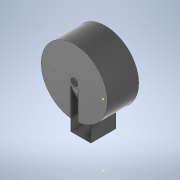
# Autodesk Inventor part: Grundplatte
Saved by Autodesk Inventor 2020.3 (Build 243373000, 373)
## iProperties
Created: 2021-08-11
Part Number: Grundplatte
Material: Acetalharz, Schwarz
Document SubType Name: Modeling
Designer: Preuß P. Ch.
Density: 1.425 g/cm^3
Appearance: Glatt - Schwarz
Author: Preuß P. Ch.
Autodesk Inventor part; units mm, degrees
ref_plane "YZ Plane" through (0, 0, 0) normal (1, 0, 0) x (0, 1, 0)
ref_plane "XZ Plane" through (0, 0, 0) normal (0, 1, 0) x (-1, 0, 0)
ref_plane "XY Plane" through (0, 0, 0) normal (0, 0, 1) x (1, 0, 0)
sketch "Skizze1" plane through (0, 0, 0) normal (0, 1, 0) x (-1, 0, 0)
  line L0 (2000, 0) -> (-2000, 0)
  line L1 (-2000, 0) -> (-2000, -10)
  line L2 (-2000, -10) -> (2000, -10)
  line L3 (2000, -10) -> (2000, 0)
  dimension "d3" = 4000
  dimension "d4" = 10
  constraints: 8 end point, 2 parallel, 1 horizontal, 1 perpendicular
  measures "d3" distance of L2.end L1.end
  measures "d4" distance of L1.end L0.end
extrude "Extrusion1" add sketch "Skizze1" along normal mid plane 4000
sketch "Skizze2" plane through (-2000, 2000, 0) normal (0, 0, 1) x (1, 0, 0)
  line L0 (20, -1975) -> (433.5, -1975)
  line L1 (433.5, -1975) -> (433.5, -2025)
  line L2 (433.5, -2025) -> (20, -2025)
  line L3 (20, -2025) -> (20, -1975)
  circle A0 centre (433.5, -1975) radius 5
  circle A1 centre (433.5, -2025) radius 5
  circle A2 centre (20, -2025) radius 5
  circle A3 centre (20, -1975) radius 5
  point P0 (2000, -2000)
  dimension "d7" = 413.5
  dimension "d8" = 50
  dimension "d9" = 10
  dimension "d10" = 10
  dimension "d11" = 10
  dimension "d12" = 10
  constraints: 8 end point, 4 centre point, 4 coincident, 2 parallel, 1 horizontal, 1 perpendicular
  measures "d7" distance of L1.end L2.end
  measures "d8" distance of L0.end L1.end
  measures "d9" diameter of A0
  measures "d10" diameter of A1
  measures "d11" diameter of A2
  measures "d12" diameter of A3
hole "Bohrung1" at (-1566.5, 25, 0) at (-1566.5, -25, 0) at (-1980, -25, 0) at (-1980, 25, 0) direction (0, 0, -1) diameter 6.647 depth 10 tip angle 118 thread size "M8x1.25" class "6H" standard "ISO Metric profile"
chamfer "Fase1" distance 1 angle 45 4 edges at (-1980, 28.3235, 0) (-1980, -21.6765, 0) (-1566.5, 28.3235, 0) (-1566.5, -21.6765, 0)
sketch "Skizze3" plane through (-2000, 2000, 0) normal (0, 0, 1) x (1, 0, 0)
  circle A0 centre (1065, -2000) radius 105
  point P0 (2000, -2000)
  dimension "d23" = 210
  constraints: 1 centre point
  measures "d23" diameter of A0
extrude "Extrusion2" cut sketch "Skizze3" against normal blind 10
chamfer "Fase2" distance 10 angle 45 1 edges at (-1040, 0, 0)
sketch "Skizze4" plane through (-2000, 2000, 0) normal (0, 0, 1) x (1, 0, 0)
  line L0 (1090, -2000) -> (1040, -2000)
  line L1 (1040, -2000) -> (1040, -1555.368)
  line L2 (1040, -1555.368) -> (1090, -1555.368)
  line L3 (1090, -1555.368) -> (1090, -2000)
  line L4 (1090, -1555.368) -> (1040, -1555.368)
  line L5 (1040, -1555.368) -> (1040, -1141.868)
  line L6 (1040, -1141.868) -> (1090, -1141.868)
  line L7 (1090, -1141.868) -> (1090, -1555.368)
  point P0 (2000, -2000)
  dimension "d29" = 50
  dimension "d30" = 444.632
  dimension "d31" = 413.5
  constraints: 16 end point, 4 parallel, 2 horizontal, 2 perpendicular, 1 point on line
  measures "d29" distance of L1.end L2.end
  measures "d30" distance of L0.end L1.end
  measures "d31" distance of L4.end L5.end
hole "Bohrung2" at (-960, 444.632, 0) at (-910, 444.632, 0) at (-960, 858.132, 0) at (-910, 858.132, 0) direction (0, 0, -1) diameter 6.647 depth 10 tip angle 118 thread size "M8x1.25" class "6H" standard "ISO Metric profile"
fillet "Rundung1" radius 0.5 1 edges at (-960, 447.9555, 0)
sketch "Skizze5" plane through (-2000, 2000, 0) normal (0, 0, 1) x (1, 0, 0)
  circle A0 centre (1065, -2000) radius 115 projected
  line L0 (715, -2155) -> (945, -2155)
  line L1 (945, -2155) -> (945, -1845)
  line L2 (945, -1845) -> (715, -1845)
  line L3 (715, -1845) -> (715, -2155)
  line L4 (715, -1845) -> (735, -1845)
  line L5 (735, -1845) -> (735, -1865)
  line L6 (735, -1865) -> (715, -1865)
  line L7 (715, -1865) -> (715, -1845)
  line L8 (945, -1845) -> (925, -1845)
  line L9 (925, -1845) -> (925, -1865)
  line L10 (925, -1865) -> (945, -1865)
  line L11 (945, -1865) -> (945, -1845)
  line L12 (945, -2155) -> (925, -2155)
  line L13 (925, -2155) -> (925, -2135)
  line L14 (925, -2135) -> (945, -2135)
  line L15 (945, -2135) -> (945, -2155)
  line L16 (715, -2155) -> (735, -2155)
  line L17 (735, -2155) -> (735, -2135)
  line L18 (735, -2135) -> (715, -2135)
  line L19 (715, -2135) -> (715, -2155)
  point P0 (2000, -2000)
  dimension "d43" = 230
  dimension "d44" = 310
  dimension "d45" = 20
  dimension "d46" = 20
  dimension "d47" = 20
  dimension "d48" = 20
  dimension "d49" = 20
  dimension "d50" = 20
  dimension "d51" = 20
  constraints: 40 end point, 10 parallel, 5 horizontal, 5 perpendicular, 1 point on line
  measures "d43" distance of L2.end L1.end
  measures "d44" distance of L1.end L0.end
  measures "d45" distance of L5.end L6.end
  measures "d46" distance of L4.end L5.end
  measures "d47" distance of L10.end L9.end
  measures "d48" distance of L13.end L14.end
  measures "d49" distance of L12.end L13.end
  measures "d50" distance of L18.end L17.end
  measures "d51" distance of L17.end L16.end
hole "Bohrung3" at (-1265, -135, 0) at (-1265, 135, 0) at (-1075, -135, 0) at (-1075, 135, 0) direction (0, 0, -1) diameter 8.376 depth 27.3 tip angle 118 thread size "M10x1.5" class "6H" standard "ISO Metric profile"
sketch "Skizze9" plane through (2000, 2000, -10) normal (0, 0, -1) x (-1, 0, 0)
  circle A0 centre (2935, -2000) radius 105 projected
  line L0 (2780, -2000) -> (2780, -2155)
  line L1 (2780, -2155) -> (2935, -2155)
  line L2 (2780, -2155) -> (3090, -2155)
  line L3 (3090, -2155) -> (3090, -1845)
  line L4 (3090, -1845) -> (2780, -1845)
  line L5 (2780, -1845) -> (2780, -2155)
  line L6 (2780, -2155) -> (2795, -2155)
  line L7 (2795, -2155) -> (2795, -2135)
  line L8 (2795, -2135) -> (2780, -2135)
  line L9 (2780, -2135) -> (2780, -2155)
  line L10 (2780, -1845) -> (2795, -1845)
  line L11 (2795, -1845) -> (2795, -1865)
  line L12 (2795, -1865) -> (2780, -1865)
  line L13 (2780, -1865) -> (2780, -1845)
  point P0 (2000, -2000)
  dimension "d73" = 155
  dimension "d74" = 310
  dimension "d75" = 310
  dimension "d76" = 15
  dimension "d77" = 20
  dimension "d78" = 20
  constraints: 28 end point, 6 parallel, 3 horizontal, 3 perpendicular, 1 point on line
  measures "d73" distance of L1.end L0.end
  measures "d74" distance of L4.end L3.end
  measures "d75" distance of L3.end L2.end
  measures "d76" distance of L8.end L7.end
  measures "d77" distance of L7.end L6.end
  measures "d78" distance of L10.end L11.end
hole "Bohrung4" at (-795, -135, -10) at (-795, 135, -10) direction (0, 0, 1) diameter 8.376 depth 27.3 tip angle 118 thread size "M10x1.5" class "6H" standard "ISO Metric profile"
chamfer "Fase3" distance 4 angle 45 2 edges at (-795, -139.188, 0) (-795, 130.812, 0)
sketch "Skizze10" plane through (-2000, 2000, 0) normal (0, 0, 1) x (1, 0, 0)
  line L0 (0, 0) -> (4000, 0) projected
  line L1 (1185, -2155) -> (943, -2155)
  line L2 (943, -2155) -> (943, -3077.5)
  line L3 (943, -3077.5) -> (1185, -3077.5)
  line L4 (1185, -3077.5) -> (1185, -2155)
  point P0 (2000, -2000)
  dimension "d92" = 242
  dimension "d93" = 922.5
  constraints: 8 end point, 2 parallel, 1 horizontal, 1 perpendicular
  measures "d92" distance of L3.end L2.end
  measures "d93" distance of L2.end L1.end
extrude "Extrusion6" cut sketch "Skizze10" against normal blind 10
sketch "Skizze11" plane through (2000, 2000, -10) normal (0, 0, -1) x (-1, 0, 0)
  line L0 (3057, -3077.5) -> (3057, -2155) projected
  line L1 (3057, -3077.5) -> (3067, -3077.5)
  line L2 (3067, -3077.5) -> (3067, -2827.5)
  line L3 (3067, -2827.5) -> (3057, -2827.5)
  line L4 (3057, -2827.5) -> (3057, -3077.5)
  line L5 (2815, -3077.5) -> (2815, -2155) projected
  line L6 (2815, -3077.5) -> (2805, -3077.5)
  line L7 (2805, -3077.5) -> (2805, -2827.5)
  line L8 (2805, -2827.5) -> (2815, -2827.5)
  line L9 (2815, -2827.5) -> (2815, -3077.5)
  line L10 (3067, -3077.5) -> (2805, -3077.5)
  line L11 (2805, -3077.5) -> (2805, -3087.5)
  line L12 (2805, -3087.5) -> (3067, -3087.5)
  line L13 (3067, -3087.5) -> (3067, -3077.5)
  point P0 (2000, -2000)
  dimension "d96" = 10
  dimension "d97" = 250
  dimension "d98" = 10
  dimension "d99" = 250
  dimension "d100" = 10
  constraints: 24 end point, 6 parallel, 3 horizontal, 3 perpendicular, 1 point on line
  measures "d96" distance of L3.end L2.end
  measures "d97" distance of L2.end L1.end
  measures "d98" distance of L7.end L8.end
  measures "d99" distance of L6.end L7.end
  measures "d100" distance of L11.end L10.end
extrude "Extrusion7" add sketch "Skizze11" along normal blind 400
sketch "Skizze12" plane through (2000, 2000, -410) normal (0, 0, -1) x (-1, 0, 0)
  line L0 (3067, -3087.5) -> (2805, -3087.5) projected
  line L1 (2805, -2827.5) -> (2805, -3087.5) projected
  line L2 (3067, -3087.5) -> (2805, -3087.5)
  line L3 (2805, -3087.5) -> (2805, -2827.5)
  line L4 (2805, -2827.5) -> (3067, -2827.5)
  line L5 (3067, -2827.5) -> (3067, -3087.5)
  point P0 (2000, -2000)
  constraints: 8 end point, 2 parallel, 1 horizontal, 1 perpendicular
extrude "Extrusion8" add sketch "Skizze12" along normal blind 10
sketch "Skizze13" plane through (-1057, -827.5, -410) normal (0, 1, 0) x (1, 0, 0)
  line L0 (252, 10) -> (-10, 10) projected
  line L1 (252, -400) -> (252, 10) projected
  line L2 (-10, 10) -> (252, 10)
  line L3 (252, 10) -> (252, -140)
  line L4 (252, -140) -> (-10, -140)
  line L5 (-10, -140) -> (-10, 10)
  point P0 (1057, -410)
  dimension "d105" = 150
  constraints: 8 end point, 2 parallel, 1 horizontal, 1 perpendicular, 1 point on line
  measures "d105" distance of L2.end L3.end
extrude "Extrusion9" add sketch "Skizze13" along normal blind 10
sketch "Skizze14" plane through (-1067, -1087.5, -10) normal (-1, 0, 0) x (0, 0, 1)
  line L0 (0, 260) -> (0, 932.5) projected
  line L1 (-260, 270) -> (0, 932.5)
  line L2 (0, 932.5) -> (0, 260)
  line L3 (0, 260) -> (-260, 260)
  line L4 (-260, 260) -> (-260, 270)
  point P0 (10, 1087.5)
  constraints: 8 end point, 2 perpendicular, 1 collinear
extrude "Extrusion10" add sketch "Skizze14" against normal blind 10
sketch "Skizze15" plane through (-805, -1087.5, -10) normal (1, 0, 0) x (0, 0, -1)
  line L0 (410, 270) -> (260, 270) projected
  line L1 (0, 932.5) -> (260, 270) projected
  line L2 (260, 270) -> (0, 932.5)
  line L3 (0, 260) -> (260, 260) projected
  line L4 (0, 932.5) -> (0, 260)
  line L5 (0, 260) -> (260, 260)
  line L6 (260, 270) -> (260, 260) projected
  line L7 (260, 260) -> (260, 270)
  point P0 (-10, 1087.5)
  constraints: 8 end point, 2 collinear, 1 perpendicular
extrude "Extrusion11" add sketch "Skizze15" against normal blind 10
sketch "Skizze16" plane through (-805, -817.5, -270) normal (0, 0.3653263, -0.9308795) x (-1, 0, 0)
  line L0 (0, 0) -> (0, 711.692525)
  line L1 (262, 711.692525) -> (262, 0)
  line L2 (0, 0) -> (262, 0)
  line L3 (262, 0) -> (262, 711.692525)
  line L4 (262, 711.692525) -> (0, 711.692525)
  line L5 (0, 711.692525) -> (0, 0)
  point P0 (-805, 859.632114)
  constraints: 8 end point, 2 parallel, 1 horizontal, 1 perpendicular
extrude "Extrusion12" add sketch "Skizze16" along normal blind 10
sketch "Skizze17" plane through (-2000, 2000, 0) normal (0, 0, 1) x (1, 0, 0)
  point P0 (2000, -2000)
sketch "Skizze18" plane through (0, -2000, 0) normal (0, -1, 0) x (1, 0, 0)
  point P0 (0, 0)
sketch "Skizze19" plane through (0, -2000, 0) normal (0, -1, 0) x (1, 0, 0)
  point P0 (0, 0)
sketch "Skizze20" plane through (2000, 2000, -10) normal (0, 0, -1) x (-1, 0, 0)
  circle A0 centre (3075, -1865) radius 4.188
  line L0 (3075, -1865) -> (2935, -1865)
  line L1 (2935, -1865) -> (2935, -2000)
  line L2 (2935, -2000) -> (3075, -2000)
  line L3 (3075, -2000) -> (3075, -1865)
  circle A1 centre (2935, -2000) radius 612.5
  circle A2 centre (2935, -2000) radius 1065
  line L4 (2805, -2151.346737) -> (2805, -2813.846737)
  line L5 (3067, -2155) -> (3067, -3087.5)
  line L6 (2805, -2598.545111) -> (3067, -2598.545111)
  line L7 (3067, -2598.545111) -> (3067, -3087.5)
  line L8 (3067, -3087.5) -> (2805, -3087.5)
  line L9 (2805, -3087.5) -> (2805, -2598.545111)
  point P0 (2000, -2000)
  point P1 (2805, -3057.03595)
  point P2 (3067, -2598.107223)
  point P3 (3067, -3056.788058)
  dimension "d117" = 1225
  dimension "d114" = 140
  dimension "d115" = 135
  constraints: 16 end point, 4 parallel, 2 horizontal, 2 perpendicular, 1 centre point, 1 coincident, 1 point on line, 3 other
  measures "d114" distance of L2.end L1.end
  measures "d115" distance of L1.end L0.end
extrude "Extrusion13" add sketch "Skizze20" along normal blind 1000 contours A1 L4 L9 A2 L5
sketch "Skizze21" plane through (2000, 2000, -420) normal (0, 0, -1) x (-1, 0, 0)
  point P0 (2000, -2000)
sketch "Skizze22" plane through (-2000, 2000, 0) normal (0, 0, 1) x (1, 0, 0)
  circle A0 centre (1065, -2000) radius 115
  arc A1 (0, -2000) -> (933, -3056.788058) centre (1065, -2000) ccw
  circle A2 centre (1065, -2000) radius 1065
  line L0 (0, -4000) -> (0, -2000)
  line L1 (4000, -4000) -> (4000, 0)
  line L2 (0, -4000) -> (4000, -4000)
  line L3 (4000, -4000) -> (4000, 0)
  line L4 (4000, 0) -> (0, 0)
  line L5 (0, 0) -> (0, -4000)
  point P0 (2000, -2000)
  constraints: 8 end point, 2 parallel, 1 coincident, 1 horizontal, 1 perpendicular, 3 other
extrude "Extrusion14" cut sketch "Skizze22" against normal blind 10 contours L5 L4 L1 L2 L0
sketch "Skizze23" plane through (2000, 2000, -420) normal (0, 0, -1) x (-1, 0, 0)
  circle A0 centre (2935, -2000) radius 115
  line L0 (3067, -3087.5) -> (3067, -3056.788058)
  circle A1 centre (2935, -2000) radius 1065
  line L1 (3067, -3087.5) -> (2805, -3087.5)
  line L2 (2805, -3057.03595) -> (2805, -2598.545111)
  line L3 (3067, -3087.5) -> (2805, -3087.5)
  line L4 (2805, -3087.5) -> (2805, -3045.983935)
  line L5 (2805, -3045.983935) -> (3067, -3045.983935)
  line L6 (3067, -3045.983935) -> (3067, -3087.5)
  point P0 (2000, -2000)
  constraints: 8 end point, 2 parallel, 1 centre point, 1 coincident, 1 horizontal, 1 perpendicular, 1 point on circle, 1 point on line
extrude "Extrusion15" cut sketch "Skizze23" against normal blind 420 contours L1 L4 A1 L0
sketch "Skizze24" plane through (2000, 2000, -420) normal (0, 0, -1) x (-1, 0, 0)
  circle A0 centre (2935, -2000) radius 115
  arc A1 (2815, -3058.217841) -> (3057, -3057.98913) centre (2935, -2000) ccw
  circle A2 centre (2935, -2000) radius 1065
  line L0 (3067, -2598.107223) -> (3067, -3056.788058)
  line L1 (3067, -2598.107223) -> (2805, -2598.107223)
  line L2 (2805, -2598.107223) -> (2805, -3086.664871)
  line L3 (2805, -3086.664871) -> (3067, -3086.664871)
  line L4 (3067, -3086.664871) -> (3067, -2598.107223)
  point P0 (2000, -2000)
  point P1 (2805, -3057.03595)
  constraints: 8 end point, 2 parallel, 1 centre point, 1 coincident, 1 horizontal, 1 perpendicular, 1 point on circle
extrude "Extrusion16" add sketch "Skizze24" along normal blind 590 contours A2 L2 L1 L0 A1
sketch "Skizze25" plane through (-1057, -827.5, -270) normal (1, 0, 0) x (0, 0, -1)
  line L0 (-270, -230.48913) -> (140, -230.48913)
  line L1 (0, 0) -> (140, -230.48913)
  line L2 (140, -230.48913) -> (140, 0)
  line L3 (140, -230.48913) -> (140, -237.5)
  line L4 (140, 0) -> (0, 0)
  point P0 (-270, 827.5)
  point P1 (140, -230.717841)
  constraints: 6 end point, 1 collinear, 1 perpendicular
extrude "Extrusion17" add sketch "Skizze25" along normal blind 242
sketch "Skizze26" plane through (-935, 0, -1010) normal (0, 0, -1) x (-1, 0, 0)
  circle A0 centre (0, 0) radius 1065
  circle A1 centre (0, 0) radius 1065
  line L0 (323.325658, -1639.734211) -> (-323.326, -1639.734211)
  line L1 (-323.326, -1639.734211) -> (-323.326, -1014.734211)
  line L2 (-323.326, -1014.734211) -> (323.325658, -1014.734211)
  line L3 (323.325658, -1014.734211) -> (323.325658, -1639.734211)
  line L4 (-323.326, -1014.734211) -> (-313.326, -1014.734211)
  line L5 (-313.326, -1024.734211) -> (313.325658, -1024.734211)
  line L6 (313.325658, -1024.734211) -> (313.325658, -1629.734211)
  line L7 (313.325658, -1629.734211) -> (-313.326, -1629.734211)
  line L8 (-313.326, -1629.734211) -> (-313.326, -1024.734211)
  point P0 (-935, 0)
  point P1 (290.077226, -1024.734211)
  point P2 (-290.077226, -1024.734211)
  point P3 (-323.325658, -1014.734211)
  dimension "d133" = 10
  constraints: 18 end point, 4 parallel, 3 horizontal, 2 perpendicular, 1 centre point
  measures "d133" distance of L4.end L5.start
extrude "Extrusion18" add sketch "Skizze26" against normal blind 800 contours A0 L5 L8 L7 L6 L3 L0 L1
sketch "Skizze27" plane through (2000, 2000, -1010) normal (0, 0, -1) x (-1, 0, 0)
  line L0 (3248.325658, -3024.734211) -> (2621.674, -3024.734211)
  line L1 (2621.674, -3024.734211) -> (2621.674, -3629.734211)
  line L2 (2621.674, -3629.734211) -> (3248.325658, -3629.734211)
  line L3 (3248.325658, -3629.734211) -> (3248.325658, -3024.734211)
  point P0 (2000, -2000)
  constraints: 8 end point, 2 parallel, 1 horizontal, 1 perpendicular
extrude "Extrusion19" add sketch "Skizze27" against normal blind 10 separate body
